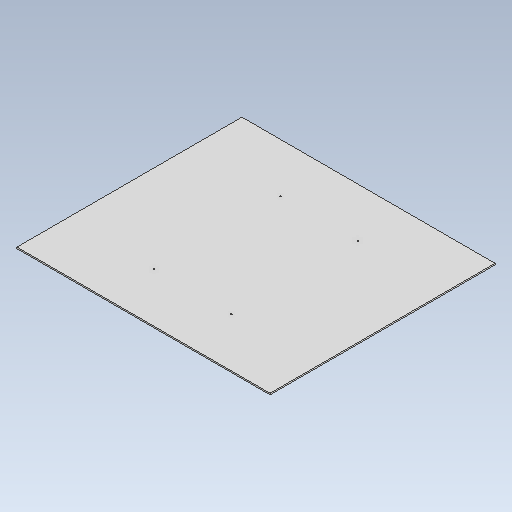
# Autodesk Inventor part: cover_base
Saved by Autodesk Inventor 2021 (Build 250183000, 183)
## iProperties
Created: 2021-05-06
Part Number: cover_base
Material: Generic
Document SubType Name: Modeling
Designer: Watchdog
Density: 1 g/cm^3
Appearance: Default
Author: Watchdog
Autodesk Inventor part; units mm, degrees
ref_plane "YZ Plane" through (0, 0, 0) normal (1, 0, 0) x (0, 1, 0)
ref_plane "XZ Plane" through (0, 0, 0) normal (0, 1, 0) x (-1, 0, 0)
ref_plane "XY Plane" through (0, 0, 0) normal (0, 0, 1) x (1, 0, 0)
sketch "Sketch1" plane through (0, 0, 0) normal (0, 1, 0) x (-1, 0, 0)
  line L0 (900, 800) -> (-900, 800)
  line L1 (-900, 800) -> (-900, -800)
  line L2 (-900, -800) -> (900, -800)
  line L3 (900, -800) -> (900, 800)
  point P0 (0, 0)
  dimension "d0" = 800
  dimension "d1" = 1600
  dimension "d2" = 1800
  dimension "d3" = 900
  constraints: 8 end point, 2 parallel, 1 horizontal, 1 perpendicular
  measures "d0" distance from line of point (0, 0) L0
  measures "d1" distance between parallel lines of L2 L0
  measures "d2" distance between parallel lines of L1 L3
  measures "d3" distance from line of point (0, 0) L3
extrude "base" add sketch "Sketch1" along normal blind 10
sketch "Sketch2" plane through (0, 10, 0) normal (0, 1, 0) x (1, 0, 0)
  point P0 (0, 0)
  point P1 (-275, -450)
  point P2 (275, -450)
  point P3 (-275, 450)
  point P4 (275, 450)
  dimension "d10" = 900
  dimension "d11" = 900
  dimension "d12" = 550
  dimension "d13" = 550
  dimension "d14" = 275
  dimension "d15" = 275
  dimension "d16" = 450
  dimension "d17" = 450
  measures "d10" distance of point (-275, 450) point (-275, -450)
  measures "d11" distance of point (275, 450) point (275, -450)
  measures "d12" distance of point (275, -450) point (-275, -450)
  measures "d13" distance of point (275, 450) point (-275, 450)
  measures "d14" horizontal distance of point (0, 0) point (-275, -450)
  measures "d15" horizontal distance of point (0, 0) point (-275, 450)
  measures "d16" vertical distance of point (0, 0) point (-275, -450)
  measures "d17" vertical distance of point (0, 0) point (275, -450)
hole "mountHoles" at (-275, 10, 450) at (275, 10, 450) at (-275, 10, -450) at (275, 10, -450) direction (0, -1, 0) diameter 10 end through all
equation "\"d0\" = 0.5 * d1"
equation "\"d1\" = cover_length_main"
equation "\"d2\" = cover_width_main"
equation "\"d3\" = 0.5 * d2"
equation "\"d4\" = cover_base_thickness"
equation "\"d10\" = cover_mountHole_xSpacing"
equation "\"d11\" = cover_mountHole_xSpacing"
equation "\"d12\" = cover_mountHole_ySpacing"
equation "\"d13\" = cover_mountHole_ySpacing"
equation "\"d14\" = 0.5 * d12"
equation "\"d15\" = 0.5 * d13"
equation "\"d16\" = 0.5 * d10"
equation "\"d17\" = 0.5 * d11"
equation "\"d18\" = cover_mountHole_diameter"
equation "\"cover_width_main\" = 1800"
equation "\"cover_length_main\" = 1600"
equation "\"cover_base_thickness\" = 10"
equation "\"cover_mountHole_diameter\" = 10"
equation "\"cover_mountHole_xSpacing\" = 900"
equation "\"cover_mountHole_ySpacing\" = 550"
equation "\"hoop_angle_z\" = 45deg"
equation "\"hoop_bearing_length\" = 5deg"
equation "\"hoop_cable_diam\" = 5"
equation "\"hoop_cable_pulley_diam\" = 22"
equation "\"rack_tooth_addendum\" = 5"
equation "\"rack_tooth_dedendum\" = 5"
equation "\"rack_tooth_thickness\" = 5"
equation "\"secure_arm_angle\" = 20deg"
equation "\"secure_arm_hold_length\" = 35"
equation "\"secure_arm_radii\" = 9"
equation "\"support_baseClamp_platformLengthBuffer\" = 35"
equation "\"support_baseClamp_platformThickness\" = 15"
equation "\"support_baseClamp_platformWidthBuffer\" = 0"
equation "\"support_baseClamp_sleeveHoleDiameter\" = 12"
equation "\"support_baseClamp_sleeveSweepTerminationAngle\" = 55deg"
equation "\"support_baseClamp_thickness\" = 8"
equation "\"support_frame_endHoleBuffer\" = 25"
equation "\"support_frame_squareBarFillet\" = 2"
equation "\"support_frame_squareBarThickness\" = 5"
body "Solid1"
